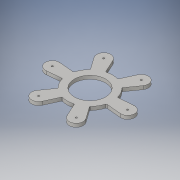
# Autodesk Inventor part: Arm Mount
Saved by Autodesk Inventor 2016 (Build 200138000, 138)
## iProperties
Created: 2016-04-16
Part Number: Arm Mount
Material: Generic
Document SubType Name: Modeling
Designer: rmarkowi
Density: 1 g/cm^3
Appearance: Default
Author: rmarkowi
Autodesk Inventor part; units mm, degrees
ref_plane "YZ Plane" through (0, 0, 0) normal (1, 0, 0) x (0, 1, 0)
ref_plane "XZ Plane" through (0, 0, 0) normal (0, 1, 0) x (-1, 0, 0)
ref_plane "XY Plane" through (0, 0, 0) normal (0, 0, 1) x (1, 0, 0)
sketch "Sketch1" plane through (0, 0, 0) normal (0, 1, 0) x (-1, 0, 0)
  circle A0 centre (0, 0) radius 57.15
  circle A1 centre (0, 0) radius 137.541 construction
  circle A2 centre (137.541, 0) radius 3.175
  circle A3 centre (68.7705, 119.114) radius 3.175
  circle A4 centre (-68.7705, 119.114) radius 3.175
  circle A5 centre (-137.541, 0) radius 3.175
  circle A6 centre (-68.7705, -119.114) radius 3.175
  circle A7 centre (68.7705, -119.114) radius 3.175
  arc A8 (89.5009, 104.4371) -> (45.6948, 129.7286) centre (68.7705, 119.114) ccw
  line L0 (45.6948, 129.7286) -> (23.6669, 81.8409)
  line L1 (89.5009, 104.4371) -> (59.0429, 61.4165)
  arc A9 (59.0429, 61.4165) -> (59.3514, 57.3752) centre (61.6342, 59.5819) ccw
  arc A10 (20.0127, 80.0874) -> (23.6669, 81.8409) centre (20.7824, 83.1677) ccw
  line L2 (-45.6948, 129.7286) -> (-23.6669, 81.8409)
  arc A11 (-23.6669, 81.8409) -> (-20.0127, 80.0874) centre (-20.7824, 83.1677) ccw
  line L3 (-89.5009, 104.4371) -> (-59.0429, 61.4165)
  arc A12 (-59.3514, 57.3752) -> (-59.0429, 61.4165) centre (-61.6342, 59.5819) ccw
  arc A13 (-45.6948, 129.7286) -> (-89.5009, 104.4371) centre (-68.7705, 119.114) ccw
  line L4 (-135.1957, 25.2915) -> (-82.7097, 20.4243)
  arc A14 (-82.7097, 20.4243) -> (-79.3641, 22.7122) centre (-82.4165, 23.5858) ccw
  line L5 (-135.1957, -25.2915) -> (-82.7097, -20.4243)
  arc A15 (-79.3641, -22.7122) -> (-82.7097, -20.4243) centre (-82.4165, -23.5858) ccw
  arc A16 (-135.1957, 25.2915) -> (-135.1957, -25.2915) centre (-137.541, 0) ccw
  line L6 (-89.5009, -104.4371) -> (-59.0429, -61.4165)
  arc A17 (-59.0429, -61.4165) -> (-59.3514, -57.3752) centre (-61.6342, -59.5819) ccw
  line L7 (-45.6948, -129.7286) -> (-23.6669, -81.8409)
  arc A18 (-20.0127, -80.0874) -> (-23.6669, -81.8409) centre (-20.7824, -83.1677) ccw
  arc A19 (-89.5009, -104.4371) -> (-45.6948, -129.7286) centre (-68.7705, -119.114) ccw
  line L8 (45.6948, -129.7286) -> (23.6669, -81.8409)
  arc A20 (23.6669, -81.8409) -> (20.0127, -80.0874) centre (20.7824, -83.1677) ccw
  line L9 (89.5009, -104.4371) -> (59.0429, -61.4165)
  arc A21 (59.3514, -57.3752) -> (59.0429, -61.4165) centre (61.6342, -59.5819) ccw
  arc A22 (45.6948, -129.7286) -> (89.5009, -104.4371) centre (68.7705, -119.114) ccw
  line L10 (135.1957, -25.2915) -> (82.7097, -20.4243)
  arc A23 (82.7097, -20.4243) -> (79.3641, -22.7122) centre (82.4165, -23.5858) ccw
  line L11 (135.1957, 25.2915) -> (82.7097, 20.4243)
  arc A24 (79.3641, 22.7122) -> (82.7097, 20.4243) centre (82.4165, 23.5858) ccw
  arc A25 (135.1957, -25.2915) -> (135.1957, 25.2915) centre (137.541, 0) ccw
  arc A26 (79.3641, 22.7122) -> (59.3514, 57.3752) centre (0, 0) ccw
  arc A27 (59.3514, -57.3752) -> (79.3641, -22.7122) centre (0, 0) ccw
  arc A28 (-20.0127, -80.0874) -> (20.0127, -80.0874) centre (0, 0) ccw
  arc A29 (-79.3641, -22.7122) -> (-59.3514, -57.3752) centre (0, 0) ccw
  arc A30 (20.0127, 80.0874) -> (-20.0127, 80.0874) centre (0, 0) ccw
  arc A31 (-59.3514, 57.3752) -> (-79.3641, 22.7122) centre (0, 0) ccw
  dimension "d0" = 114.3
  dimension "d2" = 275.082
  dimension "d3" = 6.35
  dimension "d6" = 360
  dimension "d8" = 50.8
  dimension "d9" = 6.35
  dimension "d10" = 6.35
  dimension "d13" = 360
  constraints: 52 point on circle, 32 centre point, 24 end point, 4 tangent, 3 coincident, 98 other
  measures "d0" diameter of A0
  measures "d2" diameter of A1
  measures "d3" diameter of A2
  measures "d8" diameter of A8
  measures "d9" diameter of A9
  measures "d10" diameter of A10
extrude "Extrusion1" add sketch "Sketch1" along normal blind 12.7
body "Solid1"
